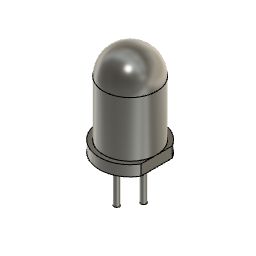
Arduino_Sequencer (Autodesk Fusion 360 archive; units mm, degrees)
design "LED_2.54mmp_D5mm"
Autodesk Fusion 360 part; units mm, degrees
sketch "スケッチ1" plane through (0, 0, 0) normal (0, 0, 1) x (1, 0, 0)
  circle A0 centre (0, 0) radius 2.9
  line L0 (2.5, 1.4697) -> (2.5, -1.4697)
  circle A1 centre (-1.27, 0) radius 0.25
  line L1 (-3.5255, 0) -> (3.8644, 0) construction
  line L2 (0, 3.5138) -> (0, -4.0944) construction
  circle A2 centre (1.27, 0) radius 0.25
  dimension "d1" = 5.8
  dimension "d8" = 2.5
  dimension "d11" = 0.5
  dimension "d14" = 1.27
  constraint coincident A0.centre origin
  constraint vertical L0
  constraint coincident A0 L0.end
  constraint coincident A0 L0.start
  constraint horizontal L1
  constraint coincident A0.centre L1
  constraint coincident A1.centre L1
  constraint vertical L2
  constraint coincident A0.centre L2
  constraint symmetric A1 L2 A2
  measures "d1" diameter of A0
  measures "d8" distance of A0.centre L0
  measures "d11" diameter of A1
  measures "d14" distance of A0.centre A1.centre
extrude "押し出し1" add sketch "スケッチ1" along normal blind 1 contours A0 L0 | A0 L0 | A1 | A2
sketch "スケッチ2" plane through (0, 0, 1) normal (0, 0, 1) x (-1, 0, 0)
  circle A0 centre (0, 0) radius 2.9
  circle A1 centre (0, 0) radius 2.5
  dimension "d4" = 5
  constraint coincident A0.centre A1.centre
  measures "d4" diameter of A1
extrude "押し出し2" add sketch "スケッチ2" along normal blind 7.7 contours A1
fillet "フィレット1" radius 2.5 1 edges at (2.3308, 0.904, 8.7)
extrude "押し出し3" cut sketch "スケッチ1" along normal blind 1 contours A0 L0 picked at (2.5576, -0.3752)
extrude "押し出し4" add sketch "スケッチ1" against normal blind 5 contours A1
extrude "押し出し5" add sketch "スケッチ1" against normal blind 3.5 contours A2

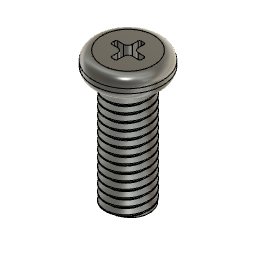
design "Screw_M3_7.5mm"
Autodesk Fusion 360 part; units mm, degrees
sketch "スケッチ1" plane through (0, 0, 0) normal (0, 0, 1) x (1, 0, 0)
  circle A0 centre (0, 0) radius 1.5
  dimension "d1" = 3
  constraint coincident A0.centre origin
  measures "d1" diameter of A0
extrude "押し出し1" add sketch "スケッチ1" along normal blind 7.5 makes body 1
thread "ねじ1" "ISO Metric profile 3.0 M3x0.5 6g" major diameter 2.927 minor diameter 2.3555 pitch 0.5 angle 60 modelled right hand crest width 0.0713 on face at (1.4925, -0.1494, 5) crest through (1.4635, 0, -0.125) on bodies 1
sketch "スケッチ2" plane through (0, 0, 7.5) normal (0, 0, 1) x (-1, 0, 0)
  spline S0 degree 3 poles (0.634, -1.319) (0.7937, -1.2229) (0.9334, -1.097) (1.1516, -0.8035) (1.2301, -0.6403) (1.317, -0.2994) (1.3272, -0.1257) (1.2801, 0.209) (1.2259, 0.367) (1.0868, 0.6046) (1.019, 0.6916) (0.864, 0.8428) (0.7781, 0.9068) (0.6847, 0.9583) knots 0 0 0 0 0.055923 0.055923 0.109803 0.109803 0.161639 0.161639 0.211432 0.211432 0.244511 0.244511 0.276632 0.276632 0.276632 0.276632
  arc A0 (0.6847, 0.9583) -> (-0.6847, 0.9583) centre (0, 0) ccw
  spline S1 degree 3 poles (-0.6847, 0.9583) (-0.821, 0.8831) (-0.941, 0.7816) (-1.1406, 0.5335) (-1.2163, 0.3878) (-1.3109, 0.0692) (-1.3263, -0.1013) (-1.2915, -0.4458) (-1.239, -0.6161) (-1.0965, -0.8832) (-1.0222, -0.9858) (-0.8463, -1.1711) (-0.7449, -1.2523) (-0.634, -1.319) knots 0 0 0 0 0.046698 0.046698 0.095434 0.095434 0.146206 0.146206 0.199015 0.199015 0.236706 0.236706 0.275362 0.275362 0.275362 0.275362
  arc A1 (-0.634, -1.319) -> (0.634, -1.319) centre (0, 0) ccw
  circle A2 centre (0, 0) radius 2.35
  dimension "d4" = 4.7
  constraint concentric A0 A2
  measures "d4" diameter of A2
extrude "押し出し2" add sketch "スケッチ2" along normal blind 1.5 separate body contours S0 A0 S1 A1 | A2 makes body 2
fillet "フィレット1" radius 0.6 2 edges at (2.191, 0.8498, 9) (2.191, 0.8498, 7.5) on bodies 2
sketch "スケッチ3" plane through (0, 0, 9) normal (0, 0, 1) x (-1, 0, 0)
  circle A0 centre (0, 0) radius 1.75
  line L0 (-1, 0) -> (-1, -0.1)
  line L1 (-0.9, -0.2) -> (-0.5, -0.2)
  line L2 (-0.2, -0.5) -> (-0.2, -0.9)
  line L3 (-0.1, -1) -> (0.1, -1)
  line L4 (0.2, -0.9) -> (0.2, -0.5)
  line L5 (0.5, -0.2) -> (0.9, -0.2)
  line L6 (1, -0.1) -> (1, 0.1)
  line L7 (0.9, 0.2) -> (0.5, 0.2)
  line L8 (0.2, 0.5) -> (0.2, 0.9)
  line L9 (0.1, 1) -> (-0.1, 1)
  line L10 (-0.2, 0.9) -> (-0.2, 0.5)
  line L11 (-0.5, 0.2) -> (-0.9, 0.2)
  line L12 (-1, 0.1) -> (-1, 0)
  arc A1 (0.5, -0.2) -> (0.2, -0.5) centre (0.5, -0.5) ccw
  arc A2 (-0.2, -0.5) -> (-0.5, -0.2) centre (-0.5, -0.5) ccw
  arc A3 (-0.5, 0.2) -> (-0.2, 0.5) centre (-0.5, 0.5) ccw
  arc A4 (0.2, 0.5) -> (0.5, 0.2) centre (0.5, 0.5) ccw
  arc A5 (0.9, -0.2) -> (1, -0.1) centre (0.9, -0.1) ccw
  arc A6 (1, 0.1) -> (0.9, 0.2) centre (0.9, 0.1) ccw
  arc A7 (0.1, -1) -> (0.2, -0.9) centre (0.1, -0.9) ccw
  arc A8 (-0.2, -0.9) -> (-0.1, -1) centre (-0.1, -0.9) ccw
  arc A9 (-1, -0.1) -> (-0.9, -0.2) centre (-0.9, -0.1) ccw
  arc A10 (-0.9, 0.2) -> (-1, 0.1) centre (-0.9, 0.1) ccw
  arc A11 (-0.1, 1) -> (-0.2, 0.9) centre (-0.1, 0.9) ccw
  arc A12 (0.2, 0.9) -> (0.1, 1) centre (0.1, 0.9) ccw
  dimension "d8" = 0.3
  dimension "d9" = 0.3
  dimension "d10" = 0.3
  dimension "d11" = 0.1
  constraint vertical L0
  constraint perpendicular L0 L1
  constraint perpendicular L1 L2
  constraint perpendicular L2 L3
  constraint perpendicular L3 L4
  constraint perpendicular L2 L5
  constraint perpendicular L3 L6
  constraint perpendicular L2 L7
  constraint perpendicular L3 L8
  constraint perpendicular L2 L9
  constraint perpendicular L9 L10
  constraint perpendicular L10 L11
  constraint perpendicular L11 L12
  constraint tangent L4 A1
  constraint tangent L5 A1
  constraint tangent L1 A2
  constraint tangent L2 A2
  constraint tangent L10 A3
  constraint tangent L11 A3
  constraint equal A2 A3
  constraint tangent L7 A4
  constraint tangent L8 A4
  constraint tangent L5 A5
  constraint tangent L6 A5
  constraint tangent L6 A6
  constraint tangent L7 A6
  constraint equal A5 A6
  constraint tangent L3 A7
  constraint tangent L4 A7
  constraint equal A5 A7
  constraint tangent L2 A8
  constraint tangent L3 A8
  constraint equal A5 A8
  constraint tangent L0 A9
  constraint tangent L1 A9
  constraint equal A5 A9
  constraint tangent L11 A10
  constraint tangent L12 A10
  constraint equal A5 A10
  constraint tangent L9 A11
  constraint tangent L10 A11
  constraint equal A5 A11
  constraint tangent L8 A12
  constraint tangent L9 A12
  constraint equal A5 A12
  measures "d8" radius of A1
  measures "d9" radius of A2
  measures "d10" radius of A4
  measures "d11" radius of A5
extrude "押し出し3" cut sketch "スケッチ3" against normal blind 1 contours L0 L1 L2 L3 L4 L5 L6 L7 L8 L9 L10 L11 L12 A1 A2 A3 A4 A5 A6 A7 A8 A9 A10 A11 A12 bodies 2

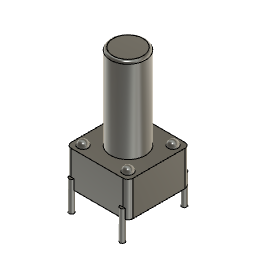
design "tactile_6x6x12"
Autodesk Fusion 360 part; units mm, degrees
sketch "スケッチ1" plane through (0, 0, 0) normal (0, 0, 1) x (1, 0, 0)
  line L0 (0, 0) -> (6.2, 0)
  line L1 (6.2, 0) -> (6.2, 6.2)
  line L2 (6.2, 6.2) -> (0, 6.2)
  line L3 (0, 6.2) -> (0, 0)
  circle A0 centre (0.56, 0) radius 0.25
  circle A1 centre (5.64, 0) radius 0.25
  line L4 (0.56, 0) -> (5.64, 0) construction
  line L5 (-0.8303, 3.1) -> (7.1697, 3.1) construction
  circle A2 centre (0.56, 6.2) radius 0.25
  circle A3 centre (5.64, 6.2) radius 0.25
  dimension "d1" = 6.2
  dimension "d2" = 6.2
  dimension "d10" = 0.5
  dimension "d11" = 5.08
  dimension "d12" = 0.56
  dimension "d13" = 3.1
  constraint horizontal L0
  constraint vertical L1
  constraint horizontal L2
  constraint vertical L3
  constraint coincident L0.start L3.end
  constraint equal A0 A1
  constraint coincident L0 A0.centre
  constraint coincident L0 A1.centre
  constraint coincident A0.centre L4.start
  constraint coincident A1.centre L4.end
  constraint perpendicular L1 L5
  constraint symmetric A0 L5 A2
  constraint symmetric A1 L5 A3
  measures "d1" distance of L0.start L0.end
  measures "d2" distance of L0.start L2.end
  measures "d10" diameter of A0
  measures "d11" distance of A0.centre A1.centre
  measures "d12" distance of L0.start A0.centre
  measures "d13" distance of L2 L5
extrude "押し出し1" add sketch "スケッチ1" along normal blind 3.5 contours L0 L1 L2 L3 A0 A1 A2 A3 | L0 A1 | L0 A0 | L2 A3 | L2 A2 picked at (5.7011, 0.0567) picked at (0.6211, 0.0567) picked at (5.588, 6.0857) picked at (0.5126, 6.0741)
sketch "スケッチ2" plane through (0, 0, 3.5) normal (0, 0, 1) x (-1, 0, 0)
  line L0 (0, -6.2) -> (0, 0)
  line L1 (0, 0) -> (-6.2, 0)
  line L2 (-6.2, 0) -> (-6.2, -6.2)
  line L3 (-6.2, -6.2) -> (0, -6.2)
  circle A0 centre (-3.1, -3.1) radius 1.75
  circle A1 centre (-0.85, -5.35) radius 0.5
  circle A2 centre (-5.35, -5.35) radius 0.5
  circle A3 centre (-5.35, -0.85) radius 0.5
  circle A4 centre (-0.85, -0.85) radius 0.5
  line L4 (0, -6.2) -> (0, 0)
  line L5 (-6.9311, -0.85) -> (1.5036, -0.85) construction
  line L6 (-0.56, 0) -> (-5.64, 0)
  line L7 (-0.85, -6.8597) -> (-0.85, 0.6131) construction
  dimension "d5" = 3.5
  dimension "d6" = 3.1
  dimension "d7" = 3.1
  dimension "d19" = 1
  dimension "d20" = 4.5
  dimension "d22" = 0.85
  dimension "d23" = 0.85
  dimension "d24" = 4.5
  dimension "d25" = 4.5
  dimension "d26" = 4.5
  constraint equal A3 A4
  constraint equal A2 A4
  constraint equal A1 A4
  constraint horizontal L5
  constraint coincident A4.centre L5
  constraint vertical L7
  constraint coincident A4.centre L7
  constraint coincident A1.centre L7
  constraint coincident A3.centre L5
  measures "d5" diameter of A0
  measures "d6" distance of L1 A0.centre
  measures "d7" distance of L0 A0.centre
  measures "d19" diameter of A4
  measures "d20" distance of A3.centre A4.centre
  measures "d22" distance of L5 L6
  measures "d23" distance of L4 L7
  measures "d24" vertical distance of A2.centre A3.centre
  measures "d25" distance of A1.centre A4.centre
  measures "d26" distance of A1.centre A2.centre
extrude "押し出し2" add sketch "スケッチ2" along normal blind 8.5 contours A0
extrude "押し出し3" add sketch "スケッチ1" against normal blind 2 contours L0 A1 | L0 A1 | L0 A0 | L0 A0 | L2 A3 | L2 A3 | L2 A2 | L2 A2
extrude "押し出し4" add sketch "スケッチ1" along normal blind 1 contours L0 A1 | L0 A0 | L2 A3 | L2 A2 picked at (5.588, -0.0652) picked at (0.4911, -0.0469) picked at (5.7011, 6.3058) picked at (0.636, 6.2486)
extrude "押し出し5" add sketch "スケッチ2" along normal blind 0.5 contours A1 | A2 | A3 | A4
fillet "フィレット1" radius 0.5 4 edges at (5.8162, 1.0308, 4) (1.3162, 1.0308, 4) (1.3162, 5.5308, 4) (5.8162, 5.5308, 4)
fillet "フィレット2" radius 0.5 4 edges at (6.2, 0, 1.75) (6.2, 6.2, 1.75) (0, 0, 1.75) (0, 6.2, 1.75)
fillet "フィレット3" radius 0.25 1 edges at (4.7316, 3.7328, 12)

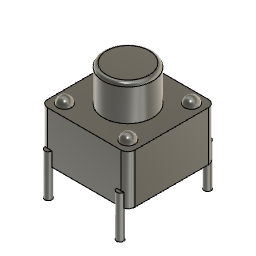
design "tactile_6x6x6"
Autodesk Fusion 360 part; units mm, degrees
sketch "スケッチ1" plane through (0, 0, 0) normal (0, 0, 1) x (1, 0, 0)
  line L0 (0, 0) -> (6.2, 0)
  line L1 (6.2, 0) -> (6.2, 6.2)
  line L2 (6.2, 6.2) -> (0, 6.2)
  line L3 (0, 6.2) -> (0, 0)
  circle A0 centre (0.56, 0) radius 0.25
  circle A1 centre (5.64, 0) radius 0.25
  line L4 (0.56, 0) -> (5.64, 0) construction
  line L5 (-0.8303, 3.1) -> (7.1697, 3.1) construction
  circle A2 centre (0.56, 6.2) radius 0.25
  circle A3 centre (5.64, 6.2) radius 0.25
  dimension "d1" = 6.2
  dimension "d2" = 6.2
  dimension "d10" = 0.5
  dimension "d11" = 5.08
  dimension "d12" = 0.56
  dimension "d13" = 3.1
  constraint horizontal L0
  constraint vertical L1
  constraint horizontal L2
  constraint vertical L3
  constraint coincident L0.start L3.end
  constraint equal A0 A1
  constraint coincident L0 A0.centre
  constraint coincident L0 A1.centre
  constraint coincident A0.centre L4.start
  constraint coincident A1.centre L4.end
  constraint perpendicular L1 L5
  constraint symmetric A0 L5 A2
  constraint symmetric A1 L5 A3
  measures "d1" distance of L0.start L0.end
  measures "d2" distance of L0.start L2.end
  measures "d10" diameter of A0
  measures "d11" distance of A0.centre A1.centre
  measures "d12" distance of L0.start A0.centre
  measures "d13" distance of L2 L5
extrude "押し出し1" add sketch "スケッチ1" along normal blind 3.5 contours L0 L1 L2 L3 A0 A1 A2 A3 | L0 A1 | L0 A0 | L2 A3 | L2 A2 picked at (5.7011, 0.0567) picked at (0.6211, 0.0567) picked at (5.588, 6.0857) picked at (0.5126, 6.0741)
sketch "スケッチ2" plane through (0, 0, 3.5) normal (0, 0, 1) x (-1, 0, 0)
  line L0 (0, -6.2) -> (0, 0)
  line L1 (0, 0) -> (-6.2, 0)
  line L2 (-6.2, 0) -> (-6.2, -6.2)
  line L3 (-6.2, -6.2) -> (0, -6.2)
  circle A0 centre (-3.1, -3.1) radius 1.75
  circle A1 centre (-0.85, -5.35) radius 0.5
  circle A2 centre (-5.35, -5.35) radius 0.5
  circle A3 centre (-5.35, -0.85) radius 0.5
  circle A4 centre (-0.85, -0.85) radius 0.5
  line L4 (0, -6.2) -> (0, 0)
  line L5 (-6.9311, -0.85) -> (1.5036, -0.85) construction
  line L6 (-0.56, 0) -> (-5.64, 0)
  line L7 (-0.85, -6.8597) -> (-0.85, 0.6131) construction
  dimension "d5" = 3.5
  dimension "d6" = 3.1
  dimension "d7" = 3.1
  dimension "d19" = 1
  dimension "d20" = 4.5
  dimension "d22" = 0.85
  dimension "d23" = 0.85
  dimension "d24" = 4.5
  dimension "d25" = 4.5
  dimension "d26" = 4.5
  constraint equal A3 A4
  constraint equal A2 A4
  constraint equal A1 A4
  constraint horizontal L5
  constraint coincident A4.centre L5
  constraint vertical L7
  constraint coincident A4.centre L7
  constraint coincident A1.centre L7
  constraint coincident A3.centre L5
  measures "d5" diameter of A0
  measures "d6" distance of L1 A0.centre
  measures "d7" distance of L0 A0.centre
  measures "d19" diameter of A4
  measures "d20" distance of A3.centre A4.centre
  measures "d22" distance of L5 L6
  measures "d23" distance of L4 L7
  measures "d24" vertical distance of A2.centre A3.centre
  measures "d25" distance of A1.centre A4.centre
  measures "d26" distance of A1.centre A2.centre
extrude "押し出し2" add sketch "スケッチ2" along normal blind 2.5 contours A0
extrude "押し出し3" add sketch "スケッチ1" against normal blind 2 contours L0 A1 | L0 A1 | L0 A0 | L0 A0 | L2 A3 | L2 A3 | L2 A2 | L2 A2
extrude "押し出し4" add sketch "スケッチ1" along normal blind 1 contours L0 A1 | L0 A0 | L2 A3 | L2 A2 picked at (5.588, -0.0652) picked at (0.4911, -0.0469) picked at (5.7011, 6.3058) picked at (0.636, 6.2486)
extrude "押し出し5" add sketch "スケッチ2" along normal blind 0.5 contours A1 | A2 | A3 | A4
fillet "フィレット1" radius 0.5 4 edges at (5.8162, 1.0308, 4) (1.3162, 1.0308, 4) (1.3162, 5.5308, 4) (5.8162, 5.5308, 4)
fillet "フィレット2" radius 0.5 4 edges at (6.2, 0, 1.75) (6.2, 6.2, 1.75) (0, 0, 1.75) (0, 6.2, 1.75)
fillet "フィレット3" radius 0.25 1 edges at (4.7316, 3.7328, 6)

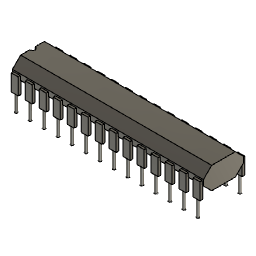
design "IC_DIP_28pin"
Autodesk Fusion 360 part; units mm, degrees
sketch "スケッチ1" plane through (0, 0, 0) normal (0, 0, 1) x (1, 0, 0)
  line L0 (-17.35, -3.65) -> (17.35, -3.65)
  line L1 (17.35, -3.65) -> (17.35, 3.65)
  line L2 (17.35, 3.65) -> (-17.35, 3.65)
  line L3 (-17.35, 3.65) -> (-17.35, -3.65)
  dimension "d1" = 34.7
  dimension "d2" = 7.3
  dimension "d23" = 17.35
  dimension "d24" = 3.65
  constraint horizontal L0
  constraint vertical L1
  constraint horizontal L2
  constraint vertical L3
  measures "d1" distance of L0.start L0.end
  measures "d2" distance of L0.start L2.end
  measures "d23" distance of origin L3
  measures "d24" distance of origin L0
extrude "押し出し1" add sketch "スケッチ1" along normal blind 4
chamfer "面取り1" distance 1.5 angle 45 4 edges at (0, -3.65, 4) (0, -3.65, 0) (0, 3.65, 4) (0, 3.65, 0)
sketch "スケッチ2" plane through (0, -3.65, 0) normal (0, -1, 0) x (1, 0, 0)
  line L0 (-17.35, 1.5) -> (17.35, 1.5)
  line L1 (17.35, 1.5) -> (17.35, 2.5)
  line L2 (17.35, 2.5) -> (-17.35, 2.5)
  line L3 (-17.35, 2.5) -> (-17.35, 1.5)
  line L4 (-17.15, 2.25) -> (-15.88, 2.25)
  line L5 (-15.88, 2.25) -> (-15.88, 1.75)
  line L6 (-15.88, 1.75) -> (-17.15, 1.75)
  line L7 (-17.15, 1.75) -> (-17.15, 2.25)
  dimension "d6" = 1.27
  dimension "d7" = 0.5
  dimension "d8" = 0.2
  dimension "d9" = 0.25
  constraint horizontal L4
  constraint vertical L5
  constraint horizontal L6
  constraint vertical L7
  measures "d6" distance of L4.start L4.end
  measures "d7" distance of L4.start L6.end
  measures "d8" distance of L3 L7
  measures "d9" distance of L0 L6
extrude "押し出し2" add sketch "スケッチ2" along normal blind 0.41 contours L4 L5 L6 L7
sketch "スケッチ3" plane through (0, 0, 1.75) normal (0, 0, -1) x (1, 0, 0)
  line L0 (-17.15, 3.65) -> (-15.88, 3.65)
  line L1 (-15.88, 3.65) -> (-15.88, 4.06)
  line L2 (-15.88, 4.06) -> (-17.15, 4.06)
  line L3 (-17.15, 4.06) -> (-17.15, 3.65)
  line L4 (-17.15, 4.06) -> (-15.88, 4.06)
  line L5 (-15.88, 4.06) -> (-15.88, 3.56)
  line L6 (-15.88, 3.56) -> (-17.15, 3.56)
  line L7 (-17.15, 3.56) -> (-17.15, 4.06)
  dimension "d12" = 0.5
  constraint horizontal L4
  constraint vertical L5
  constraint horizontal L6
  constraint vertical L7
  constraint coincident L2.end L3.start
  constraint coincident L1.end L5
  measures "d12" distance of L2.end L6.end
extrude "押し出し3" add sketch "スケッチ3" along normal blind 2.5
sketch "スケッチ4" plane through (0, 0, -0.75) normal (0, 0, -1) x (1, 0, 0)
  line L0 (-17.15, 3.56) -> (-15.88, 3.56)
  line L1 (-15.88, 3.56) -> (-15.88, 4.06)
  line L2 (-15.88, 4.06) -> (-17.15, 4.06)
  line L3 (-17.15, 4.06) -> (-17.15, 3.56)
  circle A0 centre (-16.515, 3.81) radius 0.25
  dimension "d15" = 0.5
  dimension "d16" = 0.635
  constraint tangent L2 A0
  measures "d15" diameter of A0
  measures "d16" distance of L3 A0.centre
extrude "押し出し4" add sketch "スケッチ4" along normal blind 3 contours A0
pattern_linear "R パターン1" count 14 spacing 2.54 along (1, 0, 0) of "押し出し2", "押し出し3", "押し出し4"
mirror "ミラー1" about plane through (0, 0, 0) normal (0, 1, 0) of "押し出し2", "押し出し3", "押し出し4", "R パターン1"
sketch "スケッチ5" plane through (0, 0, 4) normal (0, 0, 1) x (-1, 0, 0)
  line L0 (-17.35, -2.15) -> (17.35, -2.15)
  line L1 (17.35, -2.15) -> (17.35, 2.15)
  line L2 (17.35, 2.15) -> (-17.35, 2.15)
  line L3 (-17.35, 2.15) -> (-17.35, -2.15)
  arc A0 (17.35, 0.5) -> (17.35, -0.5) centre (17.35, 0) ccw
  line L4 (17.35, 0) -> (17.35, 0.5) construction
  line L5 (17.35, 0) -> (17.35, -0.5) construction
  dimension "d26" = 0.5
  dimension "d27" = 180
  constraint midpoint L1 A0.centre
  measures "d26" radius of A0
  measures "d27" angle of L4 L5
extrude "押し出し5" cut sketch "スケッチ5" against normal blind 0.5 contours L1 A0

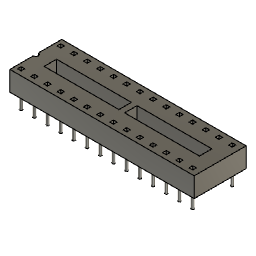
design "ICSocket_DIP28pin"
Autodesk Fusion 360 part; units mm, degrees
sketch "スケッチ1" plane through (0, 0, 0) normal (0, 0, 1) x (1, 0, 0)
  line L0 (-17.75, 5) -> (17.75, 5)
  line L1 (17.75, 5) -> (17.75, -5)
  line L2 (17.75, -5) -> (-17.75, -5)
  line L3 (-17.75, -5) -> (-17.75, 5)
  dimension "d1" = 35.5
  dimension "d2" = 10
  dimension "d3" = 17.75
  dimension "d4" = 5
  constraint horizontal L0
  constraint vertical L1
  constraint horizontal L2
  constraint vertical L3
  measures "d1" distance of L0.start L0.end
  measures "d2" distance of L0.start L2.end
  measures "d3" distance of origin L3
  measures "d4" distance of origin L0
extrude "押し出し1" add sketch "スケッチ1" along normal blind 3.8
sketch "スケッチ2" plane through (0, 0, 3.8) normal (0, 0, 1) x (-1, 0, 0)
  line L0 (17.75, 5) -> (-17.75, 5)
  line L1 (-17.75, 5) -> (-17.75, -5)
  line L2 (-17.75, -5) -> (17.75, -5)
  line L3 (17.75, -5) -> (17.75, 5)
  line L4 (-0.55, -1.2) -> (-14.95, -1.2)
  line L5 (-14.95, -1.2) -> (-14.95, 1.2)
  line L6 (-14.95, 1.2) -> (-0.55, 1.2)
  line L7 (-0.55, 1.2) -> (-0.55, -1.2)
  line L8 (14.95, -1.2) -> (0.55, -1.2)
  line L9 (0.55, -1.2) -> (0.55, 1.2)
  line L10 (0.55, 1.2) -> (14.95, 1.2)
  line L11 (14.95, 1.2) -> (14.95, -1.2)
  line L12 (0, -1.75) -> (0, -22.5)
  line L13 (17.11, 3.46) -> (16.41, 3.46)
  line L14 (16.41, 3.46) -> (16.41, 4.16)
  line L15 (16.41, 4.16) -> (17.11, 4.16)
  line L16 (17.11, 4.16) -> (17.11, 3.46)
  arc A0 (17.75, 0.5) -> (17.75, -0.5) centre (17.75, 0) ccw
  line L17 (17.75, 0) -> (17.75, 0.5) construction
  line L18 (17.75, 0) -> (17.75, -0.5) construction
  dimension "d7" = 14.4
  dimension "d8" = 2.4
  dimension "d9" = 3.8
  dimension "d10" = 2.8
  dimension "d11" = 14.4
  dimension "d12" = 2.4
  dimension "d17" = 0.7
  dimension "d18" = 0.7
  dimension "d19" = 3.46
  dimension "d20" = 0.64
  dimension "d38" = 0.5
  dimension "d39" = 180
  constraint horizontal L4
  constraint vertical L5
  constraint horizontal L6
  constraint vertical L7
  constraint horizontal L8
  constraint vertical L9
  constraint horizontal L10
  constraint vertical L11
  constraint collinear L6 L10
  constraint symmetric L7 L9 L12
  constraint horizontal L13
  constraint vertical L14
  constraint horizontal L15
  constraint vertical L16
  constraint midpoint L3 A0.centre
  measures "d7" distance of L4.start L4.end
  measures "d8" distance of L4.start L6.end
  measures "d9" distance of L0 L6
  measures "d10" distance of L1 L5
  measures "d11" distance of L8.start L8.end
  measures "d12" distance of L8.start L10.end
  measures "d17" distance of L13.start L13.end
  measures "d18" distance of L13.start L15.end
  measures "d19" distance of origin L13
  measures "d20" distance of L3 L16
  measures "d38" radius of A0
  measures "d39" angle of L17 L18
extrude "押し出し2" cut sketch "スケッチ2" against normal through all contours L3 A0 | L4 L5 L6 L7 | L8 L9 L10 L11
extrude "押し出し3" cut sketch "スケッチ2" against normal blind 3.5 contours L13 L14 L15 L16
pattern_linear "R パターン1" count 14 spacing 2.54 along (1, 0, 0) of "押し出し3"
mirror "ミラー1" about plane through (0, 0, 0) normal (0, 1, 0) of "押し出し3", "R パターン1"
sketch "スケッチ3" plane through (0, 0, 0) normal (0, 0, -1) x (1, 0, 0)
  line L0 (0.55, -1.2) -> (0.55, 1.2)
  line L1 (0.55, 1.2) -> (14.95, 1.2)
  line L2 (14.95, 1.2) -> (14.95, -1.2)
  line L3 (14.95, -1.2) -> (0.55, -1.2)
  line L4 (-14.95, -1.2) -> (-14.95, 1.2)
  line L5 (-14.95, 1.2) -> (-0.55, 1.2)
  line L6 (-0.55, 1.2) -> (-0.55, -1.2)
  line L7 (-0.55, -1.2) -> (-14.95, -1.2)
  line L8 (17.75, 5) -> (-17.75, 5)
  line L9 (-17.75, -0.5) -> (-17.75, -5)
  line L10 (-17.75, -5) -> (17.75, -5)
  line L11 (17.75, -5) -> (17.75, 5)
  line L12 (-16.41, 4.16) -> (-17.11, 4.16)
  line L13 (-16.41, 3.46) -> (-16.41, 4.16)
  line L14 (-17.11, 3.46) -> (-16.41, 3.46)
  line L15 (-17.11, 4.16) -> (-17.11, 3.46)
  circle A0 centre (-16.76, 3.81) radius 0.25
  arc A1 (-17.75, -0.5) -> (-17.75, 0.5) centre (-17.75, 0) ccw
  line L16 (-17.75, 5) -> (-17.75, 0.5)
  dimension "d28" = 0.5
  dimension "d29" = 0.35
  dimension "d30" = 0.35
  measures "d28" diameter of A0
  measures "d29" distance of L12 A0.centre
  measures "d30" distance of L15 A0.centre
extrude "押し出し4" add sketch "スケッチ3" along normal blind 3 contours A0
pattern_linear "R パターン2" count 14 spacing 2.54 along (1, 0, 0) of "押し出し4"
mirror "ミラー2" about plane through (0, 0, 0) normal (0, 1, 0) of "押し出し4", "R パターン2"

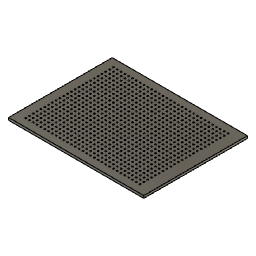
design "Universal90x70_200718_actualSize"
Autodesk Fusion 360 part; units mm, degrees
sketch "スケッチ1" plane through (0, 0, 0) normal (0, 0, 1) x (1, 0, 0)
  line L0 (0, 0) -> (90, 0)
  line L1 (90, 0) -> (90, 69)
  line L2 (90, 69) -> (0, 69)
  line L3 (0, 69) -> (0, 0)
  dimension "d1" = 90
  dimension "d2" = 69
  constraint horizontal L0
  constraint vertical L1
  constraint horizontal L2
  constraint vertical L3
  constraint coincident L0.start L3.end
  measures "d1" distance of L0.start L0.end
  measures "d2" distance of L0.start L2.end
extrude "押し出し1" add sketch "スケッチ1" along normal blind 1.6
sketch "スケッチ2" plane through (0, 0, 1.6) normal (0, 0, 1) x (-1, 0, 0)
  line L0 (0, -69) -> (0, 0)
  line L1 (0, 0) -> (-90, 0)
  line L2 (-90, 0) -> (-90, -69)
  line L3 (-90, -69) -> (0, -69)
  circle A0 centre (-6, -5.4) radius 0.5
  dimension "d5" = 1
  dimension "d6" = 5.4
  dimension "d7" = 6
  measures "d5" diameter of A0
  measures "d6" distance of L1 A0.centre
  measures "d7" distance of L0 A0.centre
extrude "押し出し2" cut sketch "スケッチ2" against normal blind 1.6 contours A0
pattern_linear "R パターン1" count 31 spacing 2.54 along (1, 0, 0) count 24 spacing 2.54 along (0, 1, 0) of "押し出し2"

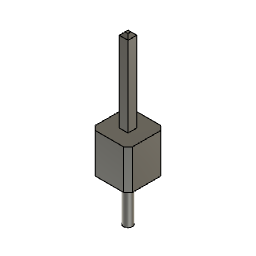
design "pinHeader_2.54mmp_1pin_Vertical"
Autodesk Fusion 360 part; units mm, degrees
sketch "スケッチ1" plane through (0, 0, 0) normal (0, 0, 1) x (1, 0, 0)
  line L0 (0, 0) -> (2.54, 0)
  line L1 (2.54, 0) -> (2.54, 2.54)
  line L2 (2.54, 2.54) -> (0, 2.54)
  line L3 (0, 2.54) -> (0, 0)
  circle A0 centre (1.27, 1.27) radius 0.3
  dimension "d1" = 2.54
  dimension "d2" = 2.54
  dimension "d12" = 0.6
  dimension "d13" = 1.27
  dimension "d14" = 1.27
  constraint horizontal L0
  constraint vertical L1
  constraint horizontal L2
  constraint vertical L3
  constraint coincident L0.start L3.end
  measures "d1" distance of L0.start L0.end
  measures "d2" distance of L0.start L2.end
  measures "d12" diameter of A0
  measures "d13" distance of L0 A0.centre
  measures "d14" distance of L3 A0.centre
extrude "押し出し1" add sketch "スケッチ1" along normal blind 2.7 contours L0 L1 L2 L3 | A0
sketch "スケッチ2" plane through (0, 0, 2.7) normal (0, 0, 1) x (-1, 0, 0)
  line L0 (0, -2.54) -> (0, 0)
  line L1 (0, 0) -> (-2.54, 0)
  line L2 (-2.54, 0) -> (-2.54, -2.54)
  line L3 (-2.54, -2.54) -> (0, -2.54)
  line L4 (-0.97, -1.57) -> (-1.57, -1.57)
  line L5 (-1.57, -1.57) -> (-1.57, -0.97)
  line L6 (-1.57, -0.97) -> (-0.97, -0.97)
  line L7 (-0.97, -0.97) -> (-0.97, -1.57)
  dimension "d5" = 0.6
  dimension "d6" = 0.6
  dimension "d7" = 0.97
  dimension "d8" = 0.97
  constraint horizontal L4
  constraint vertical L5
  constraint horizontal L6
  constraint vertical L7
  measures "d5" distance of L4.start L4.end
  measures "d6" distance of L4.start L6.end
  measures "d7" distance of L0 L7
  measures "d8" distance of L1 L6
extrude "押し出し2" add sketch "スケッチ2" along normal blind 5.7 contours L4 L5 L6 L7
chamfer "面取り1" distance 0.2 angle 45 4 edges at (1.27, 0.97, 8.4) (1.57, 1.27, 8.4) (1.27, 1.57, 8.4) (0.97, 1.27, 8.4)
extrude "押し出し3" add sketch "スケッチ1" against normal blind 3 contours A0
chamfer "面取り2" distance 0.3 angle 45 4 edges at (0, 2.54, 1.35) (0, 0, 1.35) (2.54, 0, 1.35) (2.54, 2.54, 1.35)

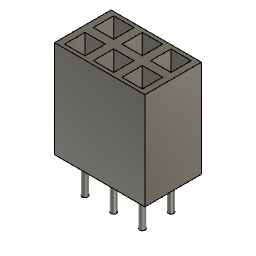
design "pinSocket_2.54mmp_2x3"
Autodesk Fusion 360 part; units mm, degrees
sketch "スケッチ1" plane through (0, 0, 0) normal (0, 0, 1) x (1, 0, 0)
  line L0 (0, 0) -> (8, 0)
  line L1 (8, 0) -> (8, 5)
  line L2 (8, 5) -> (0, 5)
  line L3 (0, 5) -> (0, 0)
  circle A0 centre (1.46, 1.23) radius 0.25
  dimension "d1" = 8
  dimension "d2" = 5
  dimension "d15" = 0.5
  dimension "d16" = 1.23
  dimension "d17" = 1.46
  constraint horizontal L0
  constraint vertical L1
  constraint horizontal L2
  constraint vertical L3
  constraint coincident L0.start L3.end
  measures "d1" distance of L0.start L0.end
  measures "d2" distance of L0.start L2.end
  measures "d15" diameter of A0
  measures "d16" distance of L0 A0.centre
  measures "d17" distance of L3 A0.centre
extrude "押し出し1" add sketch "スケッチ1" along normal blind 8.6 contours L0 L1 L2 L3 | A0
sketch "スケッチ2" plane through (0, 0, 8.6) normal (0, 0, 1) x (-1, 0, 0)
  line L0 (0, -5) -> (0, 0)
  line L1 (0, 0) -> (-8, 0)
  line L2 (-8, 0) -> (-8, -5)
  line L3 (-8, -5) -> (0, -5)
  line L4 (-0.56, -0.33) -> (-2.36, -0.33)
  line L5 (-2.36, -0.33) -> (-2.36, -2.13)
  line L6 (-2.36, -2.13) -> (-0.56, -2.13)
  line L7 (-0.56, -2.13) -> (-0.56, -0.33)
  dimension "d5" = 1.8
  dimension "d6" = 1.8
  dimension "d7" = 0.33
  dimension "d8" = 0.56
  constraint horizontal L4
  constraint vertical L5
  constraint horizontal L6
  constraint vertical L7
  measures "d5" distance of L4.start L4.end
  measures "d6" distance of L4.start L6.end
  measures "d7" distance of L1 L4
  measures "d8" distance of L0 L7
extrude "押し出し2" cut sketch "スケッチ2" against normal blind 8 contours L4 L5 L6 L7
pattern_linear "R パターン1" count 3 spacing 2.54 along (1, 0, 0) count 2 spacing 2.54 along (0, 1, 0) of "押し出し2"
extrude "押し出し3" add sketch "スケッチ1" against normal blind 3 contours A0
pattern_linear "R パターン2" count 3 spacing 2.54 along (1, 0, 0) count 2 spacing 2.54 along (0, 1, 0) of "押し出し3"
